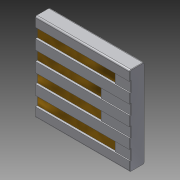
# Autodesk Inventor part: USB-Recaptacles1
Saved by Autodesk Inventor 2015 (Build 190159000, 159)
## iProperties
Created: 2021-05-13
Part Number: USB-Recaptacles1
Material: Plastic, Opaque White
Document SubType Name: Modeling
Designer: bayua
Density: 0.952 g/cm^3
Appearance: Smooth - White
Author: bayua
Autodesk Inventor part; units mm, degrees
ref_plane "YZ Plane" through (0, 0, 0) normal (1, 0, 0) x (0, 1, 0)
ref_plane "XZ Plane" through (0, 0, 0) normal (0, 1, 0) x (-1, 0, 0)
ref_plane "XY Plane" through (0, 0, 0) normal (0, 0, 1) x (1, 0, 0)
sketch "Sketch1" plane through (0, 0, 0) normal (0, 0, 1) x (1, 0, 0)
  line L0 (-6.096, 5.715) -> (6.096, 5.715)
  line L1 (6.096, 5.715) -> (6.096, -5.715)
  line L2 (6.096, -5.715) -> (-6.096, -5.715)
  line L3 (-6.096, -5.715) -> (-6.096, 5.715)
  point P0 (0, 0)
  dimension "d0" = 11.43
  dimension "d1" = 12.192
  dimension "d2" = 5.715
  dimension "d3" = 6.096
  constraints: 8 end point, 2 parallel, 1 horizontal, 1 perpendicular
  measures "d0" distance of L0.end L1.end
  measures "d1" distance of L0.start L0.end
  measures "d2" distance from line of point (0, 0) L0
  measures "d3" distance from line of point (0, 0) L3
extrude "Extrusion1" add sketch "Sketch1" along normal mid plane 1.905
sketch "Sketch2" plane through (0, 0, 0.9525) normal (0, 0, 1) x (1, 0, 0)
  line L0 (-6.096, 4.445) -> (4.064, 4.445)
  line L1 (4.064, 4.445) -> (4.064, 3.175)
  line L2 (4.064, 3.175) -> (-6.096, 3.175)
  line L3 (-6.096, 3.175) -> (-6.096, 4.445)
  line L4 (-6.096, 5.715) -> (6.096, 5.715) projected
  line L5 (-6.096, 1.905) -> (2.286, 1.905)
  line L6 (2.286, 1.905) -> (2.286, 0.635)
  line L7 (2.286, 0.635) -> (-6.096, 0.635)
  line L8 (-6.096, 0.635) -> (-6.096, 1.905)
  line L9 (-6.096, 5.715) -> (-6.096, -5.715) projected
  point P0 (0, 0)
  point P1 (-6.096, 3.81)
  point P2 (-6.096, 1.27)
  dimension "d6" = 10.16
  dimension "d7" = 1.27
  dimension "d8" = 1.27
  dimension "d9" = 1.27
  dimension "d10" = 1.27
  dimension "d11" = 8.382
  constraints: 16 end point, 4 parallel, 2 horizontal, 2 midpoint, 2 perpendicular, 1 point on line
  measures "d6" distance of L0.start L0.end
  measures "d7" distance between parallel lines of L4 L0
  measures "d8" distance of L0.end L1.end
  measures "d9" distance between parallel lines of L2 L5
  measures "d10" distance of L5.end L6.end
  measures "d11" distance of L5.start L5.end
extrude "Extrusion2" cut sketch "Sketch2" against normal blind 0.635
mirror "Mirror1" about plane through (0, 0, 0) normal (0, 1, 0) of "Extrusion2"
sketch "Sketch4" plane through (0, 0, 0.9525) normal (0, 0, 1) x (1, 0, 0)
  line L0 (1.016, 4.445) -> (6.096, 4.445)
  line L1 (6.096, 4.445) -> (6.096, 3.175)
  line L2 (6.096, 3.175) -> (1.016, 3.175)
  line L3 (1.016, 3.175) -> (1.016, 4.445)
  line L4 (-6.096, 4.445) -> (4.064, 4.445) projected
  line L5 (6.096, -5.715) -> (6.096, 5.715) projected
  point P0 (0, 0)
  dimension "d16" = 5.08
  dimension "d17" = 1.27
  constraints: 8 end point, 2 parallel, 2 point on line, 1 horizontal, 1 perpendicular
  measures "d16" distance of L0.start L0.end
  measures "d17" distance of L2.end L0.start
extrude "Extrusion3" cut sketch "Sketch4" against normal blind 0.127
pattern_linear "Rectangular Pattern1" count 4 spacing 2.54 along (0, -1, 0) of "Extrusion3"
sketch "Sketch5" plane through (0, 0, 0.3175) normal (0, 0, 1) x (1, 0, 0)
  line L0 (-6.096, 4.445) -> (4.064, 4.445)
  line L1 (4.064, 4.445) -> (4.064, 3.175)
  line L2 (4.064, 3.175) -> (-6.096, 3.175)
  line L3 (-6.096, 3.175) -> (-6.096, 4.445)
  line L4 (6.096, 0.635) -> (-6.096, 0.635) projected
  line L5 (-6.096, 1.905) -> (2.286, 1.905)
  line L6 (2.286, 1.905) -> (2.286, 0.635)
  line L7 (2.286, 0.635) -> (-6.096, 0.635)
  line L8 (-6.096, 0.635) -> (-6.096, 1.905)
  point P0 (0, 0)
  constraints: 16 end point, 4 parallel, 2 horizontal, 2 perpendicular, 1 point on line
extrude "Extrusion4" add sketch "Sketch5" along normal blind 0.381
mirror "Mirror2" about plane through (0, 0, 0) normal (0, 1, 0) of "Extrusion4"
fillet "Fillet1" radius 0.1905 4 edges at (0, -5.715, 0.9525) (0, -5.715, -0.9525) (0, 5.715, 0.9525) (0, 5.715, -0.9525)
fillet "Fillet2" radius 0.0635 24 edges at (6.096, -5.6592, -0.8967) (6.096, -5.715, 0) (6.096, -5.6592, 0.8967) (6.096, -4.9848, 0.9525) (6.096, 5.6592, -0.8967) (6.096, 5.715, 0) (6.096, 5.6592, 0.8967) (6.096, 4.9848, 0.9525) (6.096, 0, -0.9525) (6.096, -4.445, 0.889) (6.096, -3.175, 0.889) (6.096, -1.905, 0.889) (6.096, -0.635, 0.889) (6.096, 0.635, 0.889) (6.096, 1.905, 0.889) (6.096, 1.27, 0.8255) (6.096, 0, 0.9525) (6.096, -1.27, 0.8255) (6.096, -2.54, 0.9525) (6.096, -3.81, 0.8255) (6.096, 3.175, 0.889) (6.096, 4.445, 0.889) (6.096, 3.81, 0.8255) (6.096, 2.54, 0.9525)
equation "\"d2\" = 0.5 * d0"
equation "\"d3\" = 0.5 * d1"
body "Solid1"
